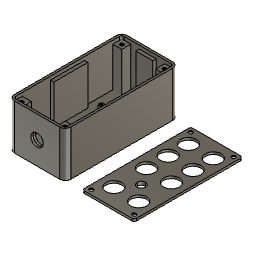
SCADD_Control_Device (Autodesk Fusion 360 design; units mm, degrees)
Autodesk Fusion 360 part; units mm, degrees
sketch "Sketch1" plane through (0, 0, 0) normal (0, 0, 1) x (1, 0, 0) in component "Box"
  line L0 (0, 0) -> (50, 0)
  line L1 (50, 0) -> (50, 100)
  line L2 (50, 100) -> (0, 100)
  line L3 (0, 100) -> (0, 0)
  line L4 (2, 2) -> (48, 2)
  line L5 (48, 2) -> (48, 98)
  line L6 (48, 98) -> (2, 98)
  line L7 (2, 98) -> (2, 2)
  line L8 (2, 98) -> (10, 98)
  line L9 (10, 98) -> (10, 90)
  line L10 (10, 90) -> (2, 90)
  line L11 (2, 90) -> (2, 98)
  line L12 (48, 98) -> (40, 98)
  line L13 (40, 98) -> (40, 90)
  line L14 (40, 90) -> (48, 90)
  line L15 (48, 90) -> (48, 98)
  line L16 (2, 2) -> (10, 2)
  line L17 (10, 2) -> (10, 10)
  line L18 (10, 10) -> (2, 10)
  line L19 (2, 10) -> (2, 2)
  line L20 (48, 2) -> (40, 2)
  line L21 (40, 2) -> (40, 10)
  line L22 (40, 10) -> (48, 10)
  line L23 (48, 10) -> (48, 2)
  circle A0 centre (6, 94) radius 1.5
  circle A1 centre (44, 94) radius 1.5
  circle A2 centre (6, 6) radius 1.5
  circle A3 centre (44, 6) radius 1.5
  line L24 (2, 65) -> (5, 65)
  line L25 (5, 65) -> (5, 35)
  line L26 (5, 35) -> (2, 35)
  line L27 (2, 35) -> (2, 65)
  line L28 (48, 35.0189) -> (45, 35.0189)
  line L29 (45, 35.0189) -> (45, 65)
  line L30 (45, 65) -> (48, 65)
  line L31 (48, 65) -> (48, 35.0189)
  line L32 (12, 70) -> (15, 70)
  line L33 (15, 70) -> (15, 67)
  line L34 (15, 67) -> (12, 67)
  line L35 (12, 67) -> (12, 70)
  line L36 (35, 70) -> (38, 70)
  line L37 (38, 70) -> (38, 67)
  line L38 (38, 67) -> (35, 67)
  line L39 (35, 67) -> (35, 70)
  line L40 (15, 20.5) -> (12, 20.5)
  line L41 (12, 20.5) -> (12, 23.5)
  line L42 (12, 23.5) -> (15, 23.5)
  line L43 (15, 23.5) -> (15, 20.5)
  line L44 (38, 20.5) -> (35, 20.5)
  line L45 (35, 20.5) -> (35, 23.5)
  line L46 (35, 23.5) -> (38, 23.5)
  line L47 (38, 23.5) -> (38, 20.5)
  line L48 (17.5, 98) -> (32.5, 98)
  line L49 (32.5, 98) -> (32.5, 95)
  line L50 (32.5, 95) -> (17.5, 95)
  line L51 (17.5, 95) -> (17.5, 98)
  line L52 (17.5, 2) -> (32.5, 2)
  line L53 (32.5, 2) -> (32.5, 4)
  line L54 (32.5, 4) -> (17.5, 4)
  line L55 (17.5, 4) -> (17.5, 2)
  line L56 (12, 69.5) -> (12, 68.5)
  line L57 (12, 68.0347) -> (11.5, 68.0347)
  line L58 (11.5, 68.0347) -> (11.5, 69.5347)
  line L59 (11.5, 69.5347) -> (12, 69.5347)
  line L60 (12, 69.5347) -> (12, 68.0347)
  line L61 (12.4991, 70) -> (14.5, 70)
  line L62 (14.5, 70) -> (14.5, 70.5)
  line L63 (14.5, 70.5) -> (12.4991, 70.5)
  line L64 (12.4991, 70.5) -> (12.4991, 70)
  line L65 (12.4654, 67) -> (14.5, 67)
  line L66 (35.4865, 70) -> (37.5, 70)
  line L67 (37.5, 70) -> (37.5, 70.5)
  line L68 (37.5, 70.5) -> (35.4865, 70.5)
  line L69 (35.4865, 70.5) -> (35.4865, 70)
  line L70 (38, 69.4972) -> (38.5, 69.4972)
  line L71 (38.5, 69.4972) -> (38.5, 67.5)
  line L72 (38.5, 67.5) -> (38, 67.5)
  line L73 (38, 67.5) -> (38, 69.4972)
  line L74 (35.503, 20.5) -> (37.5, 20.5)
  line L75 (37.5, 20.5) -> (37.5, 20)
  line L76 (37.5, 20) -> (35.503, 20)
  line L77 (35.503, 20) -> (35.503, 20.5)
  line L78 (38, 23.0037) -> (38.5, 23.0037)
  line L79 (38.5, 23.0037) -> (38.5, 21)
  line L80 (38.5, 21) -> (38, 21)
  line L81 (38, 21) -> (38, 23.0037)
  line L82 (12.5067, 20.5) -> (14.5, 20.5)
  line L83 (14.5, 20.5) -> (14.5, 20)
  line L84 (14.5, 20) -> (12.5067, 20)
  line L85 (12.5067, 20) -> (12.5067, 20.5)
  line L86 (12, 22.9913) -> (11.5, 22.9913)
  line L87 (11.5, 22.9913) -> (11.5, 21.5)
  line L88 (11.5, 21.5) -> (12, 21.5)
  line L89 (12, 21.5) -> (12, 22.9913)
  point P0 (13.5, 68.5)
  point P1 (36.5, 68.5)
  point P2 (13.5, 22)
  point P3 (36.5, 22)
  dimension "d1" = 50
  dimension "d2" = 100
  dimension "d3" = 2
  dimension "d4" = 2
  dimension "d5" = 2
  dimension "d6" = 2
  dimension "d69" = 8
  dimension "d78" = 3
  dimension "d79" = 4
  dimension "d80" = 4
  dimension "d81" = 3
  dimension "d82" = 4
  dimension "d83" = 4
  dimension "d84" = 3
  dimension "d85" = 4
  dimension "d86" = 4
  dimension "d87" = 3
  dimension "d88" = 4
  dimension "d89" = 4
  dimension "d122" = 10
  dimension "d123" = 10
  dimension "d124" = 10
  dimension "d125" = 10
  dimension "d126" = 10
  dimension "d127" = 10
  dimension "d128" = 10
  dimension "d129" = 10
  dimension "d171" = 5
  dimension "d172" = 35
  dimension "d174" = 3
  dimension "d175" = 30
  dimension "d176" = 5
  dimension "d177" = 35
  dimension "d178" = 33.0189
  dimension "d181" = 3
  dimension "d182" = 3
  dimension "d185" = 3
  dimension "d186" = 12
  dimension "d187" = 12
  dimension "d195" = 3
  dimension "d196" = 3
  dimension "d197" = 3
  dimension "d198" = 3
  dimension "d200" = 12
  dimension "d201" = 12
  dimension "d228" = 15
  dimension "d229" = 17.5
  dimension "d230" = 3
  dimension "d231" = 23
  dimension "d234" = 1.5
  dimension "d235" = 1.5
  dimension "d236" = 1.5
  dimension "d237" = 1.5
  dimension "d238" = 1.5
  dimension "d239" = 1.5
  dimension "d240" = 1.5
  dimension "d241" = 1.5
  dimension "d242" = 46.5
  dimension "d243" = 46.5
  dimension "d244" = 15
  dimension "d245" = 17.5
  dimension "d248" = 30
  dimension "d249" = 30
  dimension "d257" = 1
  dimension "d258" = 1.5
  constraint horizontal L0
  constraint vertical L1
  constraint horizontal L2
  constraint vertical L3
  constraint coincident L0.start L3.end
  constraint horizontal L4
  constraint vertical L5
  constraint horizontal L6
  constraint vertical L7
  constraint horizontal L8
  constraint vertical L9
  constraint horizontal L10
  constraint vertical L11
  constraint horizontal L12
  constraint vertical L13
  constraint horizontal L14
  constraint vertical L15
  constraint horizontal L16
  constraint vertical L17
  constraint horizontal L18
  constraint vertical L19
  constraint horizontal L20
  constraint vertical L21
  constraint horizontal L22
  constraint vertical L23
  constraint horizontal L24
  constraint vertical L25
  constraint horizontal L26
  constraint vertical L27
  constraint coincident L7 L24.start
  constraint horizontal L28
  constraint vertical L29
  constraint horizontal L30
  constraint vertical L31
  constraint coincident L5 L28.start
  constraint horizontal L32
  constraint vertical L33
  constraint horizontal L34
  constraint vertical L35
  constraint horizontal L36
  constraint vertical L37
  constraint horizontal L38
  constraint vertical L39
  constraint horizontal L40
  constraint vertical L41
  constraint horizontal L42
  constraint vertical L43
  constraint horizontal L44
  constraint vertical L45
  constraint horizontal L46
  constraint vertical L47
  constraint horizontal L48
  constraint vertical L49
  constraint horizontal L50
  constraint vertical L51
  constraint coincident L6 L48.start
  constraint horizontal L52
  constraint vertical L53
  constraint horizontal L54
  constraint vertical L55
  constraint coincident L4 L52.start
  constraint vertical L56
  constraint midpoint L35 L56.end
  constraint horizontal L57
  constraint vertical L58
  constraint horizontal L59
  constraint vertical L60
  constraint coincident L35 L57.start
  constraint horizontal L61
  constraint vertical L62
  constraint horizontal L63
  constraint vertical L64
  constraint coincident L32 L61.start
  constraint horizontal L65
  constraint coincident L34 L65.start
  constraint horizontal L66
  constraint vertical L67
  constraint horizontal L68
  constraint vertical L69
  constraint coincident L36 L66.start
  constraint horizontal L70
  constraint vertical L71
  constraint horizontal L72
  constraint vertical L73
  constraint coincident L37 L70.start
  constraint horizontal L74
  constraint vertical L75
  constraint horizontal L76
  constraint vertical L77
  constraint coincident L44 L74.start
  constraint horizontal L78
  constraint vertical L79
  constraint horizontal L80
  constraint vertical L81
  constraint coincident L47 L78.start
  constraint horizontal L82
  constraint vertical L83
  constraint horizontal L84
  constraint vertical L85
  constraint coincident L40 L82.start
  constraint horizontal L86
  constraint vertical L87
  constraint horizontal L88
  constraint vertical L89
  constraint coincident L41 L86.start
  measures "d1" distance of L0.start L0.end
  measures "d2" distance of L0.start L2.end
  measures "d3" distance of L1 L5
  measures "d4" distance of L2 L6
  measures "d5" distance of L3 L7
  measures "d6" distance of L0 L4
  measures "d69" distance of L4.start L16.end
  measures "d78" diameter of A0
  measures "d79" distance of L10 A0.centre
  measures "d80" distance of L9 A0.centre
  measures "d81" diameter of A1
  measures "d82" distance of L14 A1.centre
  measures "d83" distance of L13 A1.centre
  measures "d84" diameter of A2
  measures "d85" distance of L17 A2.centre
  measures "d86" distance of L18 A2.centre
  measures "d87" diameter of A3
  measures "d88" distance of L21 A3.centre
  measures "d89" distance of L22 A3.centre
  measures "d122" distance of L2 L10
  measures "d123" distance of L3 L9
  measures "d124" distance of L2 L14
  measures "d125" distance of L1 L13
  measures "d126" distance of L0 L22
  measures "d127" distance of L1 L21
  measures "d128" distance of L0 L18
  measures "d129" distance of L3 L17
  measures "d171" distance of L3 L25
  measures "d172" distance of L2 L24
  measures "d174" distance of L28.start L28.end
  measures "d175" distance of L24.end L25.end
  measures "d176" distance of L1 L29
  measures "d177" distance of L2 L30
  measures "d178" distance of L4.end L28
  measures "d181" distance of L32.start L32.end
  measures "d182" distance of L32.start L34.end
  measures "d185" distance of L36.end L37.end
  measures "d186" distance of L1 L37
  measures "d187" distance of L3 L35
  measures "d195" distance of L40.start L40.end
  measures "d196" distance of L40.start L42.end
  measures "d197" distance of L44.start L44.end
  measures "d198" distance of L44.start L46.end
  measures "d200" distance of L3 L41
  measures "d201" distance of L1 L47
  measures "d228" distance of L48.start L48.end
  measures "d229" distance of L3 L51
  measures "d230" distance of L36.start L36.end
  measures "d231" horizontal distance of P0 P1
  measures "d234" distance of L34 P0
  measures "d235" distance of L33 P0
  measures "d236" distance of L38 P1
  measures "d237" distance of L39 P1
  measures "d238" distance of L42 P2
  measures "d239" distance of L43 P2
  measures "d240" distance of L45 P3
  measures "d241" distance of L44 P3
  measures "d242" distance of P0 P2
  measures "d243" distance of P1 P3
  measures "d244" distance of L52.start L52.end
  measures "d245" distance of L3 L55
  measures "d248" distance of L2 L32
  measures "d249" distance of L2 L36
  measures "d257" distance of L56.end L56.start
  measures "d258" distance of L57.start L59.end
extrude "Extrude1" add sketch "Sketch1" along normal blind 40 contours L0 L1 L2 L3 makes body 1 in component "Box"
extrude "Extrude2" add sketch "Sketch1" along normal blind 2 contours L4 L7 L16 L17 L18 L19 | L4 L5 L6 L7 L9 L10 L13 L14 L17 L18 L21 L22 L24 L25 L26 L28 L29 L30 L49 L50 L51 L53 L54 L55 | L4 L52 L53 L54 L55 | L7 L24 L25 L26 L27 | L4 L5 L20 L21 L22 L23 | L6 L7 L8 L9 L10 L11 | L5 L28 L29 L30 L31 | L6 L48 L49 L50 L51 | L5 L6 L12 L13 L14 L15 | A0 | A1 | A2 | A3 | L32 L33 L34 L35 L56 L60 L61 L65 | L32 L61 L62 L63 L64 | L35 L56 L57 L58 L59 L60 | L36 L37 L38 L39 L66 L73 | L36 L66 L67 L68 L69 | L37 L70 L71 L72 L73 | L40 L41 L42 L43 L82 L89 | L40 L82 L83 L84 L85 | L41 L86 L87 L88 L89 | L44 L45 L46 L47 L74 L81 | L44 L74 L75 L76 L77 | L47 L78 L79 L80 L81 bodies 1 in component "Box"
sketch "Sketch2" plane through (0, 0, 0) normal (0, 0, 1) x (1, 0, 0) in component "Box"
  line L0 (0, 0) -> (46, 0)
  line L1 (46, 0) -> (46, 96)
  line L2 (46, 96) -> (0, 96)
  line L3 (0, 96) -> (0, 0)
  circle A0 centre (12, 82) radius 7
  circle A1 centre (34, 82) radius 7
  circle A2 centre (12, 64) radius 7
  circle A3 centre (34, 64) radius 7
  circle A4 centre (12, 45) radius 7
  circle A5 centre (34, 45) radius 7
  circle A6 centre (12, 45) radius 7
  circle A7 centre (12, 16) radius 7
  circle A8 centre (34, 16) radius 7
  spline S0 degree 3 poles (22.4434, 35) (24.1331, 35) (25.6312, 34.1799) (26.5614, 32.9159) knots 0 0 0 0 1 1 1 1
  line L4 (26.5614, 32.9159) -> (29.5871, 29.8902)
  line L5 (29.5871, 29.8902) -> (26.5614, 26.8645)
  spline S1 degree 3 poles (26.5614, 26.8645) (25.6312, 25.6006) (24.1331, 24.7805) (22.4434, 24.7805) knots 0 0 0 0 1 1 1 1
  spline S2 degree 3 poles (22.4434, 24.7805) (20.8563, 24.7805) (19.4382, 25.504) (18.501, 26.6392) knots 0 0 0 0 1 1 1 1
  line L6 (18.501, 26.6392) -> (15.25, 29.8902)
  line L7 (15.25, 29.8902) -> (18.501, 33.1413)
  spline S3 degree 3 poles (18.501, 33.1413) (19.4382, 34.2765) (20.8563, 35) (22.4434, 35) knots 0 0 0 0 1 1 1 1
  spline S4 degree 3 poles (22.4186, 26.2191) (24.4597, 26.2191) (26.1145, 27.885) (26.1145, 29.9398) knots 0 0 0 0 1 1 1 1
  spline S5 degree 3 poles (26.1145, 29.9398) (26.1145, 31.9947) (24.4597, 33.6605) (22.4186, 33.6605) knots 0 0 0 0 1 1 1 1
  spline S6 degree 3 poles (22.4186, 33.6605) (20.3774, 33.6605) (18.7227, 31.9947) (18.7227, 29.9398) knots 0 0 0 0 1 1 1 1
  spline S7 degree 3 poles (18.7227, 29.9398) (18.7227, 27.885) (20.3774, 26.2191) (22.4186, 26.2191) knots 0 0 0 0 1 1 1 1
  point P0 (4, 4)
  point P1 (4, 92)
  point P2 (42, 92)
  point P3 (42, 4)
  dimension "d130" = 46
  dimension "d131" = 96
  dimension "d144" = 4
  dimension "d145" = 4
  dimension "d146" = 4
  dimension "d147" = 4
  dimension "d148" = 4
  dimension "d149" = 4
  dimension "d150" = 4
  dimension "d151" = 4
  dimension "d267" = 14
  dimension "d268" = 12
  dimension "d269" = 14
  dimension "d270" = 14
  dimension "d271" = 14
  dimension "d272" = 12
  dimension "d273" = 14
  dimension "d274" = 14
  dimension "d275" = 12
  dimension "d276" = 12
  dimension "d277" = 32
  dimension "d278" = 32
  dimension "d279" = 14
  dimension "d280" = 14
  dimension "d281" = 12
  dimension "d282" = 12
  dimension "d283" = 51
  dimension "d284" = 51
  dimension "d287" = 14
  dimension "d288" = 14
  dimension "d289" = 12
  dimension "d290" = 14
  dimension "d291" = 12
  dimension "d292" = 80
  dimension "d293" = 80
  constraint horizontal L0
  constraint vertical L1
  constraint horizontal L2
  constraint vertical L3
  constraint coincident L0.start L3.end
  measures "d130" distance of L0.start L0.end
  measures "d131" distance of L0.start L2.end
  measures "d144" distance of L3 P0
  measures "d145" distance of L0 P0
  measures "d146" distance of L1 P2
  measures "d147" distance of L2 P2
  measures "d148" distance of L0 P3
  measures "d149" distance of L1 P3
  measures "d150" distance of L3 P1
  measures "d151" distance of L2 P1
  measures "d267" diameter of A0
  measures "d268" distance of L3 A0.centre
  measures "d269" distance of L2 A0.centre
  measures "d270" diameter of A1
  measures "d271" distance of L2 A1.centre
  measures "d272" distance of L1 A1.centre
  measures "d273" diameter of A2
  measures "d274" diameter of A3
  measures "d275" distance of L3 A2.centre
  measures "d276" distance of L1 A3.centre
  measures "d277" distance of L2 A3.centre
  measures "d278" distance of L2 A2.centre
  measures "d279" diameter of A4
  measures "d280" diameter of A5
  measures "d281" distance of L3 A4.centre
  measures "d282" distance of L1 A5.centre
  measures "d283" distance of L2 A5.centre
  measures "d284" distance of L2 A4.centre
  measures "d287" diameter of A6
  measures "d288" diameter of A7
  measures "d289" distance of L3 A7.centre
  measures "d290" diameter of A8
  measures "d291" distance of L1 A8.centre
  measures "d292" distance of L2 A8.centre
  measures "d293" distance of L2 A7.centre
extrude "Extrude1'" add sketch "Sketch1" along normal blind 37 separate body contours L6 L7 L8 L9 L10 L11 | A0 makes body 2
extrude "Extrude2'" add sketch "Sketch1" along normal blind 37 separate body contours L5 L6 L12 L13 L14 L15 | A1 makes body 3
extrude "Extrude3" add sketch "Sketch1" along normal blind 37 separate body contours L4 L5 L20 L21 L22 L23 | A3 makes body 4
extrude "Extrude4" add sketch "Sketch1" along normal blind 37 separate body contours L4 L7 L16 L17 L18 L19 | A2 makes body 5
extrude "Extrude5" cut sketch "Sketch1" along normal blind 22 and the other way blind -18 contours A0 bodies 2
extrude "Extrude6" cut sketch "Sketch1" along normal blind 22 and the other way blind -18 contours A1 bodies 3
extrude "Extrude7" cut sketch "Sketch1" along normal blind 22 and the other way blind -18 contours A2 bodies 5
extrude "Extrude8" cut sketch "Sketch1" along normal blind 22 and the other way blind -18 contours A3 bodies 4
fillet "Fillet5" radius 5 1 edges at (50, 0, 20) on bodies 1 in component "Box"
fillet "Fillet6" radius 5 1 edges at (50, 100, 20) on bodies 1 in component "Box"
fillet "Fillet7" radius 5 1 edges at (0, 100, 20) on bodies 1 in component "Box"
fillet "Fillet8" radius 5 1 edges at (0, 0, 20) on bodies 1 in component "Box"
fillet "Fillet9" radius 2 1 edges at (2, 98, 21) on bodies 1 in component "Box"
fillet "Fillet10" radius 2 1 edges at (2, 2, 21) on bodies 1 in component "Box"
fillet "Fillet11" radius 2 1 edges at (48, 2, 21) on bodies 1 in component "Box"
fillet "Fillet12" radius 2 1 edges at (48, 98, 21) on bodies 1 in component "Box"
copy_body "CutPasteBodies1" bodies 2 removing the originals makes body 6 in component "Box"
copy_body "CutPasteBodies2" bodies 3 removing the originals makes body 7 in component "Box"
copy_body "CutPasteBodies3" bodies 4 removing the originals makes body 8 in component "Box"
copy_body "CutPasteBodies4" bodies 5 removing the originals makes body 9 in component "Box"
extrude "Extrude9" add sketch "Sketch2" along normal blind 2 separate body contours L0 L1 L2 L3 | A0 | A1 | A2 | A3 | A4 A6 | A5 | A7 | A8 | S0 L4 L5 S1 S2 L6 L7 S3 | S4 S5 S6 S7 makes body 10
copy_body "CutPasteBodies5" bodies 10 removing the originals makes body 11 in component "Box"
hole "Hole1" at (4, 4, 0) at (42, 4, 0) at (4, 92, 0) at (42, 92, 0) direction (0, 0, 1) diameter 3.4 depth 2 tip angle 118 countersink diameter 6.3 countersink angle 90 bodies 11 in component "Box"
fillet "Fillet13" radius 2 1 edges at (46, 0, 1) on bodies 11 in component "Box"
fillet "Fillet14" radius 2 1 edges at (0, 0, 1) on bodies 11 in component "Box"
fillet "Fillet15" radius 2 1 edges at (46, 96, 1) on bodies 11 in component "Box"
fillet "Fillet16" radius 2 1 edges at (0, 96, 1) on bodies 11 in component "Box"
extrude "Extrude15" add sketch "Sketch1" along normal blind 37 contours L7 L24 L25 L26 L27 | L5 L28 L29 L30 L31 bodies 1 in component "Box"
extrude "Extrude10" add sketch "Sketch1" along normal blind 7 separate body contours L32 L33 L34 L35 L56 L60 L61 L65 | L36 L37 L38 L39 L66 L73 | L40 L41 L42 L43 L82 L89 | L44 L45 L46 L47 L74 L81 makes body 12 at (14, 20.5, 2.3333) makes body 13 at (37, 20.5, 2.3333) makes body 14 at (13, 70, 2.3333) makes body 15 at (36, 70, 2.3333)
hole "Hole1'" at (13.5195, 21.9848, 7) direction (0, 0, -1) diameter 1.623 depth 2 tip angle 180 bodies 12
thread "Thread1" "ISO Metric profile 2.0 M2x0.4 6H" major diameter 2.074 minor diameter 1.623 pitch 0.4 angle 60 modelled right hand crest width 0.1065 on face at (13.6003, 21.1773, 5.6667) crest through (14.331, 21.9848, 6.9) on bodies 12
hole "Hole2" at (36.5257, 21.9465, 7) direction (0, 0, -1) diameter 1.623 depth 3 tip angle 180 bodies 13
thread "Thread2" "ISO Metric profile 2.0 M2x0.4 6H" major diameter 2.074 minor diameter 1.623 pitch 0.4 angle 60 modelled right hand crest width 0.1065 on face at (36.1026, 21.254, 6) crest through (37.3372, 21.9465, 6.9) on bodies 13
hole "Hole3" at (13.5, 68.5, 7) direction (0, 0, -1) diameter 1.623 depth 3 tip angle 180 bodies 14
thread "Thread3" "ISO Metric profile 2.0 M2x0.4 6H" major diameter 2.074 minor diameter 1.623 pitch 0.4 angle 60 modelled right hand crest width 0.1065 on face at (12.7308, 68.2415, 6) crest through (14.3115, 68.5, 6.9) on bodies 14
hole "Hole4" at (36.5, 68.5, 7) direction (0, 0, -1) diameter 1.623 depth 3 tip angle 180 bodies 15
thread "Thread4" "ISO Metric profile 2.0 M2x0.4 6H" major diameter 2.074 minor diameter 1.623 pitch 0.4 angle 60 modelled right hand crest width 0.1065 on face at (35.7308, 68.2415, 6) crest through (37.3115, 68.5, 6.9) on bodies 15
hole "Hole2'" at (5.7579, 5.697, 37) direction (0, 0, -1) diameter 2.529 depth 3 tip angle 180 bodies 9 in component "Box"
thread "Thread1'" "ISO Metric profile 3.0 M3x0.5 6H" major diameter 3.086 minor diameter 2.529 pitch 0.5 angle 60 modelled right hand crest width 0.1368 on face at (5.8838, 4.4388, 35) crest through (7.0224, 5.697, 36.875) on bodies 9 in component "Box"
hole "Hole3'" at (43.9702, 5.9535, 37) direction (0, 0, -1) diameter 2.529 depth 3 tip angle 180 bodies 8 in component "Box"
thread "Thread2'" "ISO Metric profile 3.0 M3x0.5 6H" major diameter 3.086 minor diameter 2.529 pitch 0.5 angle 60 modelled right hand crest width 0.1368 on face at (44.0961, 7.2117, 36) crest through (45.2347, 5.9535, 36.875) on bodies 8 in component "Box"
hole "Hole4'" at (6.1006, 93.9457, 37) direction (0, 0, -1) diameter 2.529 depth 3 tip angle 180 bodies 6 in component "Box"
thread "Thread3'" "ISO Metric profile 3.0 M3x0.5 6H" major diameter 3.086 minor diameter 2.529 pitch 0.5 angle 60 modelled right hand crest width 0.1368 on face at (4.8459, 93.7885, 36) crest through (7.3651, 93.9457, 36.875) on bodies 6 in component "Box"
hole "Hole5" at (43.7523, 94.0551, 37) direction (0, 0, -1) diameter 2.529 depth 3 tip angle 180 bodies 7 in component "Box"
thread "Thread4'" "ISO Metric profile 3.0 M3x0.5 6H" major diameter 3.086 minor diameter 2.529 pitch 0.5 angle 60 modelled right hand crest width 0.1368 on face at (42.4976, 93.8979, 36) crest through (45.0168, 94.0551, 36.875) on bodies 7 in component "Box"
copy_body "CutPasteBodies6" bodies 12 13 14 15 removing the originals makes body 16 makes body 17 makes body 18 makes body 19 in component "Box"
extrude "Extrude16" add sketch "Sketch1" along normal blind 37 contours L6 L48 L49 L50 L51 bodies 1 in component "Box"
extrude "Extrude11" add sketch "Sketch1" along normal blind 37 separate body contours L4 L52 L53 L54 L55 makes body 20
hole "Hole5'" at (25, 0, 20) direction (0, 1, 0) diameter 11 depth 5 tip angle 118 bodies 20
hole "Hole6" at (25, 0, 20) direction (0, 1, 0) diameter 11 depth 5 tip angle 118 bodies 1 in component "Box"
extrude "Extrude17" add sketch "Sketch1" along normal blind 7 contours L32 L61 L62 L63 L64 | L35 L56 L57 L58 L59 L60 bodies 1 18 in component "Box"
extrude "Extrude18" add sketch "Sketch1" along normal blind 7 contours L36 L66 L67 L68 L69 | L37 L70 L71 L72 L73 bodies 1 19 in component "Box"
extrude "Extrude12" add sketch "Sketch1" along normal blind 7 separate body contours L40 L82 L83 L84 L85 | L41 L86 L87 L88 L89 makes body 21 at (13.8356, 20, 2.3333) makes body 22 at (12, 21.9971, 2.3333)
extrude "Extrude13" add sketch "Sketch1" along normal blind 7 separate body contours L44 L74 L75 L76 L77 | L47 L78 L79 L80 L81 makes body 23 at (36.8343, 20, 2.3333) makes body 24 at (38, 22.3358, 2.3333)
extrude "Extrude19" cut sketch "Sketch2" along normal blind 13 contours A0 | A1 | A2 | A3 | A4 A6 | A5 bodies 11 in component "Box"
extrude "Extrude20" cut sketch "Sketch2" along normal blind 23 contours A7 | A8 bodies 11 in component "Box"
extrude "Extrude23" cut sketch "Sketch2" along normal blind 39 contours S4 S5 S6 S7 bodies 11 in component "Box"
extrude "Extrude24" add sketch "Sketch2" against normal blind 1 contours S0 L4 L5 S1 S2 L6 L7 S3 bodies 11 in component "Box"
move_body "Move3" bodies 11 to x (1, 0, 0) y (0, 1, 0) z (0, 0, 1) at (65, 0, 0) in component "Box"
copy_body "CutPasteBodies7" bodies 20 21 22 23 24 removing the originals makes body 25 makes body 26 makes body 27 makes body 28 makes body 29 in component "Box"
component "Box" placed x (1, 0, 0) y (0, 1, 0) z (0, 0, 1) at (0, 0, 0)
